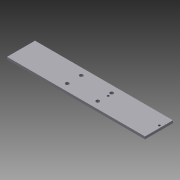
# Autodesk Inventor part: Battery Board
Saved by Autodesk Inventor 2012 (Build 160160000, 160)
## iProperties
Created: 2012-04-02
Part Number: Battery Board
Material: Aluminum-6061
Document SubType Name: Modeling
Designer: Jaime
Density: 2.71 g/cm^3
Mass: 52.9831 g
Surface Area: 138.864 cm^2
Volume: 19.551 cm^3
Author: Jaime
Autodesk Inventor part; units mm, degrees
ref_plane "YZ Plane" through (0, 0, 0) normal (1, 0, 0) x (0, 1, 0)
ref_plane "XZ Plane" through (0, 0, 0) normal (0, 1, 0) x (-1, 0, 0)
ref_plane "XY Plane" through (0, 0, 0) normal (0, 0, 1) x (1, 0, 0)
sketch "Sketch1" plane through (0, 0, 0) normal (0, 0, 1) x (1, 0, 0)
  line L0 (0, 0) -> (175.26, 0)
  line L1 (175.26, 0) -> (175.26, -35.56)
  line L2 (175.26, -35.56) -> (0, -35.56)
  line L3 (0, -35.56) -> (0, 0)
  dimension "d0" = 175.26
  dimension "d1" = 35.56
  constraints: 8 end point, 2 parallel, 1 horizontal, 1 perpendicular
  measures "d0" distance of L0.start L0.end
  measures "d1" distance of L2.end L0.start
extrude "Extrusion1" add sketch "Sketch1" along normal blind 3.175
sketch "Sketch7" plane through (0, 0, 3.175) normal (0, 0, 1) x (1, 0, 0)
  line L0 (0, 0) -> (175.26, 0) projected
  line L1 (175.26, -35.56) -> (0, -35.56) projected
  line L2 (111.125, 1.27) -> (111.125, -35.56)
  line L3 (111.125, 1.27) -> (101.6, 1.27)
  line L4 (101.6, -35.56) -> (101.6, 1.27)
  line L5 (111.125, -35.56) -> (101.6, -35.56)
  line L6 (62.865, 1.27) -> (62.865, -35.56)
  line L7 (62.865, -35.56) -> (72.39, -35.56)
  line L8 (72.39, -35.56) -> (72.39, 1.27)
  line L9 (62.865, 1.27) -> (72.39, 1.27)
  circle A0 centre (106.3625, -26.67) radius 1.651
  circle A1 centre (106.3625, -8.89) radius 1.651
  point P0 (67.6275, -8.89)
  point P1 (67.6275, -26.67)
  point P2 (106.3625, -8.89)
  point P3 (106.3625, -26.67)
  dimension "d97" = 26.67
  dimension "d98" = 8.89
  dimension "d99" = 8.89
  dimension "d100" = 26.67
  dimension "d101" = 8.89
  constraints: 16 end point, 2 centre point
  measures "d97" distance from line of L1 point (67.627, -8.89)
  measures "d98" distance from line of L1 point (67.627, -26.67)
  measures "d99" distance from line of L0 point (67.627, -8.89)
  measures "d100" distance from line of L1 point (106.362, -8.89)
  measures "d101" distance from line of L1 point (106.362, -26.67)
hole "Hole5" at (67.6275, -8.89, 3.175) at (67.6275, -26.67, 3.175) at (106.3625, -8.89, 3.175) at (106.3625, -26.67, 3.175) direction (0, 0, -1) diameter 4.4958 end through all clearance for "Hex Machine Screw" size "#8" standard "Ansi Unified Screw Threads"
sketch "Sketch8" plane through (0, 0, 3.175) normal (0, 0, 1) x (1, 0, 0)
  arc A0 (172.26, -12.306) -> (172.26, -16.306) centre (172.26, -14.306) ccw projected
  arc A1 (107.26, -16.306) -> (107.26, -12.306) centre (107.26, -14.306) ccw projected
  constraints: 2 coincident
hole "Hole6" at (107.26, -14.306, 3.175) at (172.26, -14.306, 3.175) direction (0, 0, -1) diameter 2.6416 end through all thread size "6-32 UNC" class "2B" standard "ANSI Unified Screw Threads"
body "Solid1"
